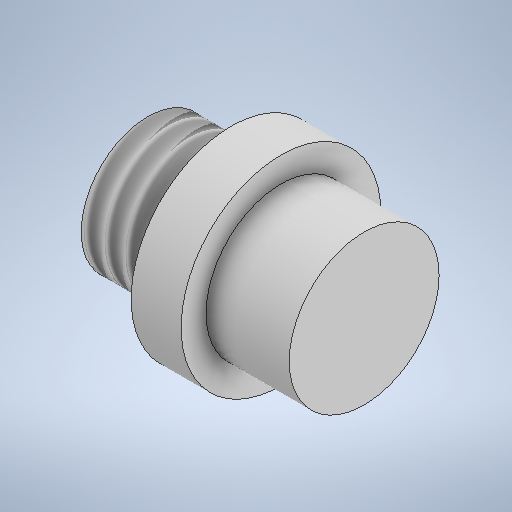
# Autodesk Inventor part: 139
Saved by Autodesk Inventor 2025.1 (Build 291241000, 241)
## iProperties
Created: 2024-08-05
Part Number: 139
Material: Generisch
Document SubType Name: Modeling
Designer: ffogue
Density: 1 g/cm^3
Appearance: Vorgabe
Author: ffogue
Autodesk Inventor part; units mm, degrees
ref_plane "YZ Plane" through (0, 0, 0) normal (1, 0, 0) x (0, 1, 0)
ref_plane "XY Plane" through (0, 0, 0) normal (0, 0, 1) x (1, 0, 0)
sketch "Sketch1" plane through (0, 0, 0) normal (0, 0, 1) x (1, 0, 0)
  line L0 (0, 0) -> (0, 4)
  line L1 (0, 4) -> (5, 4)
  line L2 (5, 4) -> (5, 6)
  line L3 (5, 6) -> (8, 6)
  line L4 (8, 6) -> (8, 4.5)
  line L5 (8, 4.5) -> (13, 4.5)
  line L6 (13, 4.5) -> (13, 0)
  line L7 (13, 0) -> (0, 0)
  dimension "d0" = 9
  dimension "d1" = 8
  dimension "d2" = 5
  dimension "d3" = 5
  dimension "d4" = 3
  dimension "d5" = 12
  constraints: 16 end point, 7 perpendicular, 1 vertical
  measures "d0" diameter of L5 L7
  measures "d1" diameter of L1 L7
  measures "d2" distance of L4.end L5.end
  measures "d3" distance of L0.end L1.end
  measures "d4" distance of L2.end L3.end
  measures "d5" diameter of L3 L7
revolve "Revolution1" add sketch "Sketch1" angle 360 about axis through (13, 0, 0) along (-1, 0, 0)
thread "Thread1" size "M8x1.25" class "6g" standard "ISO Metric profile" length 10
body "Solid1"
